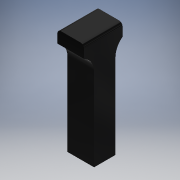
# Autodesk Inventor part: frontside arm
Saved by Autodesk Inventor 2019 (Build 230136000, 136)
## iProperties
Created: 2019-10-24
Part Number: frontside arm
Material: UHMW, Black
Document SubType Name: Modeling
Designer: robgr
Density: 0.94 g/cm^3
Appearance: Smooth - Black
Mass: 7.10736 g
Surface Area: 36.0763 cm^2
Volume: 7.56102 cm^3
Author: robgr
Autodesk Inventor part; units mm, degrees
ref_plane "YZ Plane" through (0, 0, 0) normal (1, 0, 0) x (0, 1, 0)
ref_plane "XZ Plane" through (0, 0, 0) normal (0, 1, 0) x (-1, 0, 0)
ref_plane "XY Plane" through (0, 0, 0) normal (0, 0, 1) x (1, 0, 0)
sketch "Sketch1" plane through (0, 0, 0) normal (0, 0, 1) x (1, 0, 0)
  circle A0 centre (0, 0) radius 2
  line L0 (-5.5, 3.5) -> (5.5, 3.5)
  line L1 (7.5, 1.5) -> (7.5, -3.5)
  line L2 (7.5, -3.5) -> (-7.5, -3.5)
  line L3 (-7.5, -3.5) -> (-7.5, 1.5)
  arc A1 (-5.5, 3.5) -> (-7.5, 1.5) centre (-5.5, 1.5) ccw
  arc A2 (7.5, 1.5) -> (5.5, 3.5) centre (5.5, 1.5) ccw
  point P0 (7.5, 3.5)
  dimension "d0" = 4
  dimension "d1" = 15
  dimension "d2" = 7
  dimension "d3" = 7.5
  dimension "d4" = 3.5
  dimension "d5" = 2
  constraints: 8 end point, 4 point on circle, 4 tangent, 3 centre point, 2 parallel, 2 point on line, 1 coincident, 1 equal radius, 1 horizontal, 1 perpendicular
  measures "d0" diameter of A0
  measures "d1" distance of L1.end L2.end
  measures "d2" distance of point (7.5, 3.5) L1.end
  measures "d3" distance from line of L3 point (0, 0)
  measures "d4" distance from line of L2 point (0, 0)
  measures "d5" radius of A1
extrude "Extrusion1" add sketch "Sketch1" against normal blind 16
sketch "Sketch2" plane through (-7.5, -3.5, 0) normal (0, -1, 0) x (-1, 0, 0)
  line L0 (-15, 0) -> (-13, 0) projected
  line L1 (0, 12) -> (-15, 12)
  line L2 (-15, 12) -> (-15, 0)
  line L3 (-15, 0) -> (0, 0)
  line L4 (0, 0) -> (0, 12)
  line L5 (-15, 16) -> (0, 16) projected
  line L6 (0, 0) -> (0, 16) projected
  point P0 (-7.5, 0)
  dimension "d8" = 4
  dimension "d9" = 0
  dimension "d18" = 15
  dimension "d19" = 12
  constraints: 8 end point, 2 parallel, 1 horizontal, 1 perpendicular
  measures "d8" distance between parallel lines of L5 L1
  measures "d9" distance between parallel lines of L6 L4
  measures "d18" distance of L0.start L3.end
  measures "d19" distance between parallel lines of L3 L1
extrude "Extrusion2" add sketch "Sketch2" along normal blind 55.5
fillet "Fillet2" radius 10 1 edges at (0, -3.5, -12)
sketch "Sketch4" plane through (0, 0, 0) normal (0, 0, 1) x (1, 0, 0)
  line L0 (7.5, -3.5) -> (-7.5, -3.5) projected
  line L1 (7.5, -3.5) -> (-7.5, -3.5)
  line L2 (-7.5, -3.5) -> (-7.5, 1.5)
  line L3 (-5.5, 3.5) -> (5.5, 3.5)
  line L4 (7.5, 1.5) -> (7.5, -3.5)
  arc A0 (-5.5, 3.5) -> (-7.5, 1.5) centre (-5.5, 1.5) ccw
  arc A1 (7.5, 1.5) -> (5.5, 3.5) centre (5.5, 1.5) ccw
  point P0 (0, 0)
  dimension "d14" = 2
  constraints: 8 end point, 4 point on circle, 4 tangent, 2 centre point, 2 parallel, 1 equal radius, 1 horizontal, 1 perpendicular
  measures "d14" radius of A0
extrude "Extrusion3" add sketch "Sketch4" along normal blind 5.6
fillet "Fillet3" radius 10 1 edges at (0, -3.5, 0)
body "Solid1"
